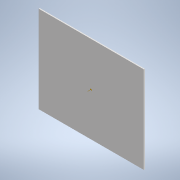
# Autodesk Inventor part: панель_с_электроникой
Saved by Autodesk Inventor 2021.1 (Build 251245010, 245A)
## iProperties
Created: 2023-01-21
Part Number: панель_с_электроникой
Material: Типовые
Document SubType Name: ЛистМат
Designer: zmoze
Density: 1 g/cm^3
Sheet Metal Rule: По умолчанию_мм
Appearance: По умолчанию
Author: zmoze
Autodesk Inventor part; units mm, degrees
ref_plane "YZ Plane" through (0, 0, 0) normal (1, 0, 0) x (0, 1, 0)
ref_plane "XZ Plane" through (0, 0, 0) normal (0, 1, 0) x (-1, 0, 0)
ref_plane "XY Plane" through (0, 0, 0) normal (0, 0, 1) x (1, 0, 0)
sketch "Эскиз1" plane through (0, 0, 0) normal (0, 0, 1) x (1, 0, 0)
  line L0 (-145, 120) -> (145, 120)
  line L1 (145, 120) -> (145, -120)
  line L2 (145, -120) -> (-145, -120)
  line L3 (-145, -120) -> (-145, 120)
  line L4 (-145, 120) -> (145, -120) construction
  line L5 (145, 120) -> (-145, -120) construction
  point P0 (0, 0)
  dimension "d0" = 240
  dimension "d1" = 290
  measures "d0" distance of L2.end L0.start
  measures "d1" distance of L0.start L0.end
extrude "Пластина1" add sketch "Эскиз1" along normal blind 3
sketch "Эскиз2" plane through (0, 0, 3) normal (0, 0, 1) x (1, 0, 0)
  line L0 (12.5, 105) -> (-12.5, 105) projected
  line L1 (-12.5, 105) -> (-12.5, 115) projected
  line L2 (-12.5, 115) -> (12.5, 115) projected
  line L3 (12.5, 115) -> (12.5, 105) projected
  line L4 (122, -15.0105) -> (122, 14.9895) projected
  line L5 (122, 14.9895) -> (132, 14.9895) projected
  line L6 (132, 14.9895) -> (132, -15.0105) projected
  line L7 (132, -15.0105) -> (122, -15.0105) projected
  line L8 (122.0074, 94.9791) -> (132.0074, 94.9783) projected
  line L9 (132.0074, 94.9783) -> (132.0051, 64.9783) projected
  line L10 (132.0051, 64.9783) -> (122.0051, 64.9791) projected
  line L11 (122.0051, 64.9791) -> (122.0074, 94.9791) projected
  line L12 (12.5, -105) -> (12.5, -115) projected
  line L13 (12.5, -115) -> (-12.5, -115) projected
  line L14 (-12.5, -115) -> (-12.5, -105) projected
  line L15 (-12.5, -105) -> (12.5, -105) projected
  circle A0 centre (-107, 95) radius 1.5 projected
  circle A1 centre (107, -95) radius 1.5 projected
  circle A2 centre (107, 95) radius 1.5 projected
  line L16 (122, -65) -> (132, -65) projected
  line L17 (132, -65) -> (132, -95) projected
  line L18 (132, -95) -> (122, -95) projected
  line L19 (122, -95) -> (122, -65) projected
  circle A3 centre (-107, -95) radius 1.5 projected
  line L20 (-147, 125) -> (-147, -125) projected
  line L21 (-147, -125) -> (147, -125) projected
  line L22 (147, -125) -> (147, 125) projected
  line L23 (147, 125) -> (-147, 125) projected
  point P0 (0, 0)
extrude "Выдавливание1" cut sketch "Эскиз2" against normal through all contours L0 L1 L2 L3 | L4 L5 L6 L7 | L8 L9 L10 L11 | L12 L13 L14 L15 | A0 | A1 | A2 | L16 L17 L18 L19 | A3
equation "\"d2\" = Толщина"
equation "\"Радиус_гибки\" = Толщина"
equation "\"Ширина_просечки\" = Толщина"
equation "\"Глубина_просечки\" = 0.5 * Толщина"
equation "\"Размер_просечки\" = 4 * Толщина"
equation "\"Мин_остаток\" = 2 * Толщина"
equation "\"Радиус_перехода\" = Радиус_гибки"
equation "\"Радиус_Якоби\" = Радиус_гибки"
equation "\"Размер_зазора\" = Толщина"
equation "\"Толщина\" = 3"
